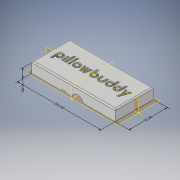
# Autodesk Inventor part: top
Saved by Autodesk Inventor 2019 (Build 230136000, 136)
## iProperties
Created: 2019-08-09
Part Number: top
Material: Generic
Document SubType Name: Modeling
Designer: tmst0
Density: 1 g/cm^3
Appearance: Default
Author: tmst0
Autodesk Inventor part; units mm, degrees
sketch "Sketch8" plane through (0, 0, 0) normal (0, 1, 0) x (-1, 0, 0)
  line L0 (101.5, -46.5) -> (-101.5, -46.5)
  line L1 (-101.5, -46.5) -> (-101.5, 46.5)
  line L2 (-101.5, 46.5) -> (101.5, 46.5)
  line L3 (101.5, 46.5) -> (101.5, -46.5)
  line L4 (101.5, -46.5) -> (-101.5, 46.5) construction
  line L5 (-101.5, -46.5) -> (101.5, 46.5) construction
  point P0 (0, 0)
  dimension "d19" = 203
  dimension "d20" = 93
  constraints: 12 end point, 2 midpoint, 2 parallel, 1 horizontal, 1 perpendicular
  measures "d19" distance of L1.end L2.end
  measures "d20" distance of L0.end L1.end
extrude "Extrusion4" add sketch "Sketch8" along normal blind 26
shell "Shell3" thickness 3 removed faces 1 at (-33.8333, 0, -15.5)
sketch "Sketch11" plane through (0, 0, 0) normal (0, 1, 0) x (-1, 0, 0)
  line L0 (-100, 45) -> (100, 45)
  line L1 (100, 45) -> (100, -45)
  line L2 (100, -45) -> (-100, -45)
  line L3 (-100, -45) -> (-100, 45)
  line L4 (-100, 45) -> (100, -45) construction
  line L5 (100, 45) -> (-100, -45) construction
  point P0 (0, 0)
  dimension "d28" = 200
  dimension "d29" = 90
  constraints: 12 end point, 2 midpoint, 2 parallel, 1 horizontal, 1 perpendicular
  measures "d28" distance of L1.end L2.end
  measures "d29" distance of L0.end L1.end
extrude "Extrusion6" cut sketch "Sketch11" along normal blind 5
sketch "Sketch12" plane through (0, 26, 0) normal (0, 1, 0) x (1, 0, 0)
  arc A0 (-83.0974, -6.8353) -> (-81.9257, -7.3904) centre (-79.0974, 0.0929) ccw
  line L0 (-87.0974, 0.0929) -> (-87.0974, -0.7936)
  line L1 (-87.0974, -15.9071) -> (-83.0974, -14.9071)
  line L2 (-83.0974, -14.9071) -> (-83.0974, -7.9214)
  line L3 (-67.9549, 7.0929) -> (-63.9549, 7.981)
  line L4 (-67.9549, 7.0929) -> (-67.9549, -7.9071)
  line L5 (-67.9549, -7.9071) -> (-63.9549, -7.9071)
  line L6 (-63.9549, -7.9071) -> (-63.9549, 7.981)
  line L7 (-61.0356, 15.1386) -> (-57.0356, 16.0722)
  line L8 (-61.0356, 15.1386) -> (-61.0356, 0.1386)
  line L9 (-57.0356, 0.1386) -> (-57.0356, 16.0722)
  line L10 (-28.0974, 8.06) -> (-24.0974, 8.06)
  line L11 (-24.0974, 8.06) -> (-22.0974, 0.0929)
  line L12 (-22.0974, 0.0929) -> (-20.0974, 8.06)
  line L13 (-20.0974, 8.06) -> (-16.0974, 8.06)
  line L14 (-16.0974, 8.06) -> (-14.0974, 0.0929)
  line L15 (-14.0974, 0.0929) -> (-12.0974, 8.06)
  line L16 (-12.0974, 8.06) -> (-8.0974, 8.06)
  line L17 (-8.0974, 8.06) -> (-12.4291, -7.9071)
  line L18 (-12.4291, -7.9071) -> (-16.4291, -7.9071)
  line L19 (-16.4291, -7.9071) -> (-18.0974, 0.0764)
  line L20 (-18.0974, 0.0764) -> (-20.0891, -7.9071)
  line L21 (-20.0891, -7.9071) -> (-24.0974, -7.8741)
  line L22 (-24.0974, -7.8741) -> (-28.0974, 8.06)
  line L23 (-4.0995, 0.076) -> (-4.0974, 2.5929)
  line L24 (49.9026, 16.0929) -> (45.9026, 15.0929)
  line L25 (45.9026, 15.0929) -> (45.9026, 8.0353)
  arc A1 (34.2224, -2.1464) -> (49.6429, -1.9291) centre (41.9026, 0.0929) ccw
  arc A2 (38.0214, -0.8744) -> (45.5839, 1.6577) centre (41.9026, 0.0929) ccw
  line L26 (49.9026, 0.0929) -> (49.9026, 2.5786)
  line L27 (-0.0974, 16.1318) -> (-0.0974, 7.0095)
  arc A3 (10.7911, 4.1511) -> (3.0681, 8.0373) centre (3.9026, 0.0786) ccw
  line L28 (64.9026, 15.0929) -> (64.9026, 9.542)
  line L29 (68.9026, 16.0929) -> (64.9026, 15.0929)
  line L30 (68.9026, 0.0929) -> (68.9026, 3.1038)
  line L31 (-53.0974, 15.1647) -> (-49.0974, 16.1318)
  line L32 (-53.0974, 15.1647) -> (-53.0974, 0.1647)
  line L33 (-49.0974, 0.1647) -> (-49.0974, 16.1318)
  line L34 (64.9026, 9.542) -> (64.9026, 7.0211)
  line L35 (64.5839, 1.6577) -> (64.9026, 1.7645)
  arc A4 (57.0214, -0.8744) -> (64.713, -1.124) centre (60.9026, 0.0929) ccw
  arc A5 (53.2224, -2.1464) -> (60.9026, -7.9071) centre (60.9026, 0.0929) ccw
  arc A6 (64.713, -1.124) -> (64.9026, 0.0929) centre (60.9026, 0.0929) ccw
  arc A7 (64.9026, -6.8353) -> (68.9026, 0.0929) centre (60.9026, 0.0929) ccw
  arc A8 (60.9026, -7.9071) -> (64.9026, -6.8353) centre (60.9026, 0.0929) ccw
  line L36 (68.9026, 4.5196) -> (68.9026, 8.0353)
  line L37 (56.9243, 0.5089) -> (52.9549, -0.8202)
  line L38 (53.2224, -2.1464) -> (57.0214, -0.8744)
  line L39 (68.9026, 4.5196) -> (67.7978, 4.1496)
  line L40 (68.3828, 2.9297) -> (68.9026, 3.1038)
  line L41 (64.9026, 1.7645) -> (68.3828, 2.9297)
  arc A9 (63.8284, 2.8206) -> (56.9243, 0.5089) centre (60.9026, 0.0929) ccw
  line L42 (67.7978, 4.1496) -> (63.8284, 2.8206)
  arc A10 (64.9026, 0.0929) -> (64.5839, 1.6577) centre (60.9026, 0.0929) ccw
  line L43 (68.9026, 8.0353) -> (68.9026, 16.0929)
  arc A11 (64.9026, 7.0211) -> (52.9549, -0.8202) centre (60.9026, 0.0929) ccw
  arc A12 (-76.2032, 2.854) -> (-83.0706, 0.5546) centre (-79.0974, 0.0929) ccw
  line L44 (-75.4327, 1.6962) -> (-71.6321, 2.9687)
  line L45 (-72.224, 4.1864) -> (-76.2032, 2.854)
  line L46 (-83.0974, -7.3808) -> (-83.0974, -6.8353)
  arc A13 (-82.9886, -0.8337) -> (-75.4327, 1.6962) centre (-79.0974, 0.0929) ccw
  arc A14 (-72.224, 4.1864) -> (-73.4542, 5.7634) centre (-79.0974, 0.0929) ccw
  line L47 (-87.0974, -2.2094) -> (-87.0974, -5.9071)
  line L48 (-87.0974, -2.2094) -> (-86.7892, -2.1062)
  line L49 (-87.0974, -5.9071) -> (-87.0974, -15.9071)
  line L50 (-83.0974, -7.9214) -> (-83.0974, -7.3808)
  arc A15 (-81.9257, -7.3904) -> (-76.3925, -7.4359) centre (-79.0974, 0.0929) ccw
  line L51 (-83.0706, 0.5546) -> (-83.0974, 0.5457)
  arc A16 (-76.3925, -7.4359) -> (-71.6321, 2.9687) centre (-79.0974, 0.0929) ccw
  arc A17 (-73.4542, 5.7634) -> (-86.7077, 2.5592) centre (-79.0974, 0.0929) ccw
  line L52 (-87.0499, -0.7777) -> (-87.0974, -0.7936)
  line L53 (-86.7892, -2.1062) -> (-83.0974, -0.8701)
  line L54 (-83.0974, 0.5457) -> (-87.0499, -0.7777)
  line L55 (-83.0974, -0.8701) -> (-82.9886, -0.8337)
  arc A18 (-86.7077, 2.5592) -> (-87.0974, 0.0929) centre (-79.0974, 0.0929) ccw
  line L56 (-34.0666, 1.5648) -> (-30.2677, 2.8368)
  arc A19 (-41.6291, -0.9673) -> (-34.0666, 1.5648) centre (-37.7478, 0) ccw
  arc A20 (-34.8221, 2.7276) -> (-41.7261, 0.416) centre (-37.7478, 0) ccw
  arc A21 (-30.8527, 4.0567) -> (-45.6955, -0.9131) centre (-37.7478, 0) ccw
  line L57 (-30.8527, 4.0567) -> (-34.8221, 2.7276)
  arc A22 (-45.428, -2.2393) -> (-30.2677, 2.8368) centre (-37.7478, 0) ccw
  line L58 (-45.428, -2.2393) -> (-41.6291, -0.9673)
  line L59 (-41.7261, 0.416) -> (-45.6955, -0.9131)
  line L60 (-0.0765, 0.5094) -> (-0.0974, 0.5024)
  line L61 (7.5785, 1.6559) -> (11.3775, 2.9293)
  arc A23 (6.8191, 2.8197) -> (-0.0765, 0.5094) centre (3.9026, 0.0786) ccw
  arc A24 (0.0181, -0.8755) -> (0.0839, -1.1118) centre (3.9026, 0.0786) ccw
  arc A25 (7.8323, 0.8253) -> (7.5785, 1.6559) centre (3.9026, 0.0786) ccw
  line L62 (10.7911, 4.1511) -> (6.8191, 2.8197)
  arc A26 (-3.781, -2.1489) -> (-0.0974, -6.8496) centre (3.9026, 0.0786) ccw
  arc A27 (-4.0995, 0.076) -> (-4.0486, -0.822) centre (3.9026, 0.0786) ccw
  line L63 (-4.0974, 5.0929) -> (-4.0974, 15.1647)
  line L64 (-4.0974, 2.5929) -> (-4.0974, 5.0929)
  arc A28 (3.0681, 8.0373) -> (-0.0974, 7.0095) centre (3.9026, 0.0786) ccw
  arc A29 (11.7161, 1.7963) -> (11.3775, 2.9293) centre (3.9026, 0.0786) ccw
  arc A30 (4.3803, -7.9071) -> (11.7161, 1.7963) centre (3.9026, 0.0786) ccw
  arc A31 (0.0839, -1.1118) -> (7.8323, 0.8253) centre (3.9026, 0.0786) ccw
  line L65 (-3.781, -2.1489) -> (0.0181, -0.8755)
  line L66 (-0.0974, 0.5024) -> (-4.0486, -0.822)
  arc A32 (-0.0974, -6.8496) -> (4.3803, -7.9071) centre (3.9026, 0.0786) ccw
  line L67 (37.9243, 0.5089) -> (33.9549, -0.8202)
  arc A33 (44.8284, 2.8206) -> (37.9243, 0.5089) centre (41.9026, 0.0929) ccw
  line L68 (45.5839, 1.6577) -> (49.9026, 3.1038)
  line L69 (48.7978, 4.1496) -> (44.8284, 2.8206)
  line L70 (49.9026, 4.5196) -> (49.9026, 8.0353)
  line L71 (49.9026, 4.5196) -> (48.7978, 4.1496)
  arc A34 (45.9026, 7.0211) -> (42.8611, 8.0353) centre (41.9026, 0.0929) ccw
  line L72 (45.9026, 8.0353) -> (45.9026, 7.0211)
  line L73 (49.9026, 8.0353) -> (49.9026, 16.0929)
  arc A35 (42.8611, 8.0353) -> (33.9549, -0.8202) centre (41.9026, 0.0929) ccw
  line L74 (34.2224, -2.1464) -> (38.0214, -0.8744)
  line L75 (49.9026, 2.5786) -> (49.9026, 3.1038)
  arc A36 (49.6429, -1.9291) -> (49.9026, 0.0929) centre (41.9026, 0.0929) ccw
  line L76 (72.2725, 7.981) -> (76.2725, 7.981)
  line L77 (76.2725, 7.981) -> (79.6408, -2.2301)
  line L78 (79.6408, -2.2301) -> (83.097, 7.981)
  line L79 (83.097, 7.981) -> (87.097, 7.981)
  line L80 (87.097, 7.981) -> (78.98, -16)
  line L81 (78.98, -16) -> (74.98, -16)
  line L82 (72.2725, 7.981) -> (77.4051, -7.5788)
  line L83 (-4.0974, 15.1647) -> (-0.0974, 16.1318)
  arc A37 (18.9726, -0.0193) -> (26.9726, -0.0193) centre (22.9726, -0.0193) ccw
  line L84 (26.9726, -0.0193) -> (26.9726, 6.9089)
  line L85 (26.9726, 7.9807) -> (30.9726, 7.9807)
  line L86 (30.9726, 7.9807) -> (30.9726, 6.6104)
  line L87 (18.9726, -0.0193) -> (18.9726, 6.9089)
  line L88 (18.9726, 7.9807) -> (14.9726, 7.9807)
  line L89 (14.9726, 7.9807) -> (14.9726, 4.1371)
  line L90 (26.9726, 6.9089) -> (26.9726, 7.9807)
  line L91 (18.9726, 6.9089) -> (18.9726, 7.9807)
  arc A38 (14.9726, -0.0193) -> (17.8917, -6.1986) centre (22.9726, -0.0193) ccw
  line L92 (30.9726, 6.6104) -> (30.9726, -0.0193)
  line L93 (14.9726, 4.1371) -> (14.9726, -0.0193)
  arc A39 (17.8917, -6.1986) -> (30.1749, -3.5016) centre (22.9726, -0.0193) ccw
  arc A40 (30.1749, -3.5016) -> (30.9726, -0.0193) centre (22.9726, -0.0193) ccw
  line L94 (-61.0356, -7.9071) -> (-57.0356, -7.9071)
  line L95 (-61.0356, 0.1386) -> (-61.0356, -7.9071)
  line L96 (-57.0356, 0.1386) -> (-57.0356, -7.9071)
  line L97 (-53.0974, -7.9071) -> (-49.0974, -7.9071)
  line L98 (-53.0974, 0.1647) -> (-53.0974, -7.9071)
  line L99 (-49.0974, 0.1647) -> (-49.0974, -7.9071)
  line L100 (-101.5, 46.5) -> (-101.5, -46.5) projected
  line L101 (101.5, -46.5) -> (101.5, 46.5) projected
  line L102 (74.98, -16) -> (77.4051, -7.5788)
  line L103 (101.5, 46.5) -> (-101.5, 46.5) projected
  point P0 (3.9026, 0.0786)
  point P1 (-57.0356, 0.6048)
  point P2 (-49.0974, 0.6977)
  dimension "d39" = 4
  dimension "d40" = 4
  dimension "d46" = 4
  dimension "d54" = 4
  dimension "d63" = 4
  dimension "d64" = 4
  dimension "d82" = 14.4026
  dimension "d83" = 14.403
  dimension "d84" = 22.52
  dimension "d85" = 38.519
  dimension "d86" = 38.5192
  dimension "d87" = 38.519
  dimension "d88" = 38.519
  constraints: 202 end point, 85 point on circle, 74 parallel, 41 centre point, 34 tangent, 28 point on line, 14 vertical, 7 horizontal, 6 coincident, 5 perpendicular
  measures "d39" distance of L4.end L5.end
  measures "d40" distance of L8.end L9.start
  measures "d46" distance of L17.end L18.end
  measures "d54" distance of L32.end L33.start
  measures "d63" distance of L76.start L76.end
  measures "d64" distance of L78.end L79.end
  measures "d82" distance between parallel lines of L100 L47
  measures "d83" distance from line of L101 L79.end
  measures "d84" distance from line of L101 L80.end
  measures "d85" distance between parallel lines of L103 L79
  measures "d86" distance between parallel lines of L103 L85
  measures "d87" distance between parallel lines of L103 L76
  measures "d88" distance from line of L103 L3.end
extrude "Extrusion7" cut sketch "Sketch12" along normal mid plane 10
fillet "Fillet1" radius 3 4 edges at (0, 26, 46.5) (101.5, 26, 0) (0, 26, -46.5) (-101.5, 26, 0)
sketch "Sketch13" plane through (-101.5, 0, 46.5) normal (0, 0, 1) x (1, 0, 0)
  circle A0 centre (111.5, -3) radius 14
  circle A1 centre (78.5, -8) radius 11.5
  line L0 (203, 0) -> (203, 23) projected
  line L1 (-40.6, 0) -> (243.6, 0) projected
  point P0 (101.5, 0)
  dimension "d74" = 28
  dimension "d75" = 23
  dimension "d76" = 124.5
  dimension "d77" = 91.5
  dimension "d78" = 3
  dimension "d79" = 8
  constraints: 2 centre point
  measures "d74" diameter of A0
  measures "d75" diameter of A1
  measures "d76" distance from line of L0 A1.centre
  measures "d77" distance from line of L0 A0.centre
  measures "d78" distance from line of L1 A0.centre
  measures "d79" distance from line of L1 A1.centre
extrude "Extrusion8" cut sketch "Sketch13" against normal blind 10
body "Solid4"
